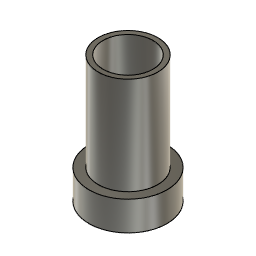
BloopSpool01 (Autodesk Fusion 360 design; units mm, degrees)
Autodesk Fusion 360 part; units mm, degrees
sketch "Sketch1" plane through (0, 0, 0) normal (0, 0, 1) x (1, 0, 0) in component "SpoolBottom"
  circle A0 centre (0, 0) radius 6.35
  dimension "d49" = 12.7
  constraint coincident A0.centre origin
  measures "d49" diameter of A0
extrude "Extrude1" add sketch "Sketch1" along normal blind 4.7625 in component "SpoolBottom"
sketch "Sketch2" plane through (0, 0, 4.7625) normal (0, 0, 1) x (-1, 0, 0) in component "SpoolBottom"
  circle A0 centre (0, 0) radius 6.35
  circle A1 centre (0, 0) radius 4.8617
  dimension "d52" = 9.7234
  constraint concentric A0 A1
  measures "d52" diameter of A1
extrude "Extrude2" add sketch "Sketch2" along normal blind 15.875 contours A1 in component "SpoolBottom"
sketch "Sketch3" plane through (0, 0, 20.6375) normal (0, 0, 1) x (-1, 0, 0) in component "SpoolBottom"
  circle A0 centre (0, 0) radius 4.8617
  circle A1 centre (0, 0) radius 4.068
  dimension "d55" = 8.1359
  constraint coincident A0.centre A1.centre
  measures "d55" diameter of A1
extrude "Extrude3" cut sketch "Sketch3" against normal blind 21.59 contours A1 in component "SpoolBottom"
chamfer "Chamfer1" distance 0.3969 angle 45 1 edges at (3.7927, 1.471, 0) in component "SpoolBottom"
sketch "Sketch4" plane through (0, 0, 4.7625) normal (0, 0, 1) x (-1, 0, 0) in component "SpoolBottom"
  circle A0 centre (0, 0) radius 4.8617
  circle A1 centre (0, 0) radius 6.35
  line L0 (5.0818, 0.2586) -> (6.5041, 0.2586)
  line L1 (6.5041, 0.2586) -> (6.5041, -0.2527)
  line L2 (6.5041, -0.2527) -> (5.0818, -0.2527)
  line L3 (5.0818, -0.2527) -> (5.0818, 0.2586)
  constraint horizontal L0
  constraint vertical L1
  constraint horizontal L2
  constraint vertical L3
extrude "Extrude4" cut sketch "Sketch4" against normal blind 4.826 contours A1 L0 L2 L3 picked at (5.5046, 0.002) in component "SpoolBottom"
component "SpoolBottom" placed x (1, 0, 0) y (0, 1, 0) z (0, 0, 1) at (0, 0, 0)
equation "d50 = ( 3 / 16 ) * 1 in"
equation "d52 = ( 5 / 16 ) * 1 in + ( 1 / 128 ) * 1 in + ( 2 / 32 ) * 1 in"
equation "d53 = ( 5 / 8 ) * 1 in"
equation "d55 = ( 5 / 16 ) * 1 in + ( 1 / 128 ) * 1 in"
equation "d58 = ( 1 / 64 ) * 1 in"
